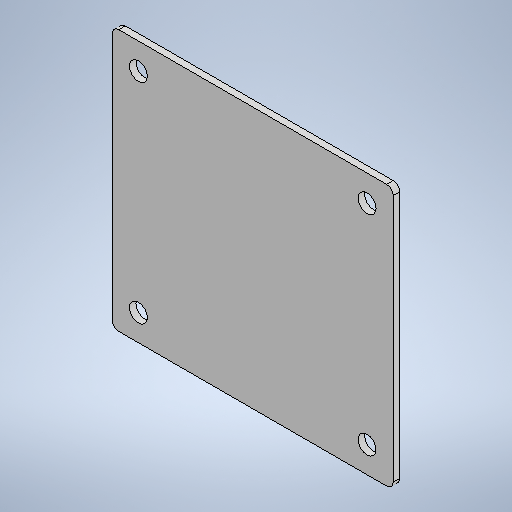
# Autodesk Inventor part: NDM 7.47 bracket floor pillar
Saved by Autodesk Inventor 2025 (Build 290162010, 162A)
## iProperties
Part Number: NDM 7.47 bracket floor pillar
Flat Pattern Width: 8.6 cm
Flat Pattern Length: 8 cm
Flat Pattern Area: 68.8 cm^2
Sheet Metal Rule: Default_mm
Sheet Metal Width: 86,000 mm
Sheet Metal Length: 80,000 mm
Sheet Metal Area: 6880,000 mm^2
Autodesk Inventor part; units mm, degrees
ref_plane "YZ Plane" through (0, 0, 0) normal (1, 0, 0) x (0, 1, 0)
ref_plane "XZ Plane" through (0, 0, 0) normal (0, 1, 0) x (-1, 0, 0)
ref_plane "XY Plane" through (0, 0, 0) normal (0, 0, 1) x (1, 0, 0)
sketch "Sketch13" plane through (0, 0, 0) normal (0, 0, 1) x (1, 0, 0)
  line L0 (-43, -40) -> (-43, 40)
  circle A0 centre (-35, 32) radius 2.75
  circle A1 centre (-35, -32) radius 2.75
  line L1 (-43, 40) -> (43, 40)
  line L2 (43, 40) -> (43, -40)
  line L3 (43, -40) -> (-43, -40)
  line L4 (0, 40) -> (0, -40) construction
  line L5 (-20, 40) -> (-20, -40) construction
  line L6 (20, 40) -> (20, -40) construction
  line L7 (-43, 0) -> (43, 0) construction
  circle A2 centre (35, 32) radius 2.75
  circle A3 centre (35, -32) radius 2.75
  line L8 (20, 40) -> (-18, 40)
  line L9 (20, -40) -> (-10, -40)
  point P0 (0, 0)
  point P1 (40, 0)
  point P2 (0, 0)
  dimension "d96" = 80
  dimension "d100" = 5.5
  dimension "d101" = 8
  dimension "d106" = 40
  dimension "d107" = 8
  dimension "d111" = 23
  measures "d96" distance of L0.start L0.end
  measures "d100" diameter of A0
  measures "d101" distance from line of A0.centre L0
  measures "d106" distance between parallel lines of L5 L6
  measures "d107" distance from line of A0.centre L1
  measures "d111" distance between parallel lines of L5 L0
extrude "Plate6" add sketch "Sketch13" along normal blind 2
fillet "Fillet4" radius 2 4 edges at (43, 40, 1) (-43, 40, 1) (-43, -40, 1) (43, -40, 1)
equation "\"d108\" = Thickness"
equation "\"BendRadius\" = Thickness"
equation "\"BendReliefWidth\" = Thickness"
equation "\"BendReliefDepth\" = 0.5 * Thickness"
equation "\"CornerReliefSize\" = 4 * Thickness"
equation "\"MinimumRemnant\" = 2 * Thickness"
equation "\"TransitionRadius\" = BendRadius"
equation "\"JacobiRadiusSize\" = BendRadius"
equation "\"GapSize\" = Thickness"
equation "\"Thickness\" = 2"
body "Solid3"
